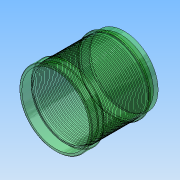
# Autodesk Inventor part: Signal_tower_D
Saved by Autodesk Inventor 2017.3 (Build 213256000, 256)
## iProperties
Created: 2017-03-21
Part Number: Signal_tower_D
Material: Polykarbonát, Čirý
Document SubType Name: Modeling
Designer: CAD
Mass: 43.1519 g
Surface Area: 356.955 cm^2
Volume: 35.9599 cm^3
Density: 1.2 g/cm^3
Appearance: LED – zelená – zap.
Stock Number: SIEMENS
Hmotnost: 0
Hotovo: 0
Objem: 0
X: 0
Y: 0
Z: 0
Author: CAD
Autodesk Inventor part; units mm, degrees
ref_plane "YZ Plane" through (0, 0, 0) normal (1, 0, 0) x (0, 1, 0)
ref_plane "XZ Plane" through (0, 0, 0) normal (0, 1, 0) x (-1, 0, 0)
ref_plane "XY Plane" through (0, 0, 0) normal (0, 0, 1) x (1, 0, 0)
sketch "Náčrt2" plane through (0, 0, 0) normal (0, 0, 1) x (1, 0, 0)
  line L0 (0, 0) -> (-32.5, 0) construction
  line L1 (-32.5, 0) -> (-32.5, 9)
  line L2 (-32.5, 9) -> (-31, 9)
  line L3 (-31, 9) -> (-31, 63)
  line L4 (0, 0) -> (0, 63) construction
  line L5 (-32.5, 0) -> (-35, 0)
  line L6 (-35, 0) -> (-35, 12)
  line L7 (-35, 12) -> (-33, 12)
  line L8 (-33, 12) -> (-33, 55)
  line L9 (-33, 55) -> (-34.5, 55)
  line L10 (-34.5, 55) -> (-34.5, 57)
  line L11 (-34.5, 57) -> (-32.5, 57)
  line L12 (-32.5, 57) -> (-32.5, 66)
  line L13 (-32.5, 66) -> (0, 66)
  line L14 (0, 66) -> (0, 63)
  line L15 (0, 63) -> (-31, 63)
  dimension "d0" = 65
  dimension "d1" = 9
  dimension "d2" = 62
  dimension "d3" = 70
  dimension "d4" = 12
  dimension "d5" = 66
  dimension "d6" = 55
  dimension "d7" = 2
  dimension "d8" = 66
  dimension "d9" = 65
  dimension "d10" = 3
  dimension "d11" = 69
  dimension "d12" = 9
  constraints: 32 end point, 7 perpendicular, 5 horizontal, 4 vertical
  measures "d0" diameter of L1 L4
  measures "d1" distance between parallel lines of L2 L0
  measures "d2" diameter of L3 L4
  measures "d3" diameter of L6 L4
  measures "d4" distance between parallel lines of L7 L5
  measures "d5" diameter of L8 L4
  measures "d6" distance between parallel lines of L9 L0
  measures "d7" distance between parallel lines of L11 L9
  measures "d8" distance between parallel lines of L13 L5
  measures "d9" diameter of L12 L4
  measures "d10" distance between parallel lines of L15 L13
  measures "d11" diameter of L10 L4
  measures "d12" distance between parallel lines of L11 L13
revolve "Rotace1" add sketch "Náčrt2" angle 360 about axis through (0, 0, 0) along (0, 1, 0)
sketch "Náčrt3" plane through (0, 0, 0) normal (0, 0, 1) x (1, 0, 0)
  circle A0 centre (-33.25, 14.5) radius 0.75
  line L0 (35, 12) -> (-35, 12) projected
  line L1 (34.5, 55) -> (-34.5, 55) projected
  line L2 (0, -11) -> (0, 66) projected
  line L3 (-32.5, 16.4967) -> (-32.5, 12.9176) construction
  line L4 (0, 0) -> (0, -18.5925) construction
  circle A1 centre (-33.25, 17) radius 0.75
  circle A2 centre (-33.25, 19.5) radius 0.75
  circle A3 centre (-33.25, 22) radius 0.75
  circle A4 centre (-33.25, 24.5) radius 0.75
  circle A5 centre (-33.25, 27) radius 0.75
  circle A6 centre (-33.25, 29.5) radius 0.75
  circle A7 centre (-33.25, 32) radius 0.75
  circle A8 centre (-33.25, 34.5) radius 0.75
  circle A9 centre (-33.25, 37) radius 0.75
  circle A10 centre (-33.25, 39.5) radius 0.75
  circle A11 centre (-33.25, 42) radius 0.75
  circle A12 centre (-33.25, 44.5) radius 0.75
  circle A13 centre (-33.25, 47) radius 0.75
  circle A14 centre (-33.25, 49.5) radius 0.75
  circle A15 centre (-33.25, 52) radius 0.75
  dimension "d14" = 1.5
  dimension "d15" = 2.5
  dimension "d28" = 65
  dimension "d31" = 2.5
  constraints: 16 centre point, 4 end point, 2 vertical, 1 point on line, 1 tangent, 30 other
  measures "d14" diameter of A0
  measures "d15" distance from line of A0.centre L0
  measures "d28" diameter of L3 L4
  measures "d31" distance of A0.centre A1.centre
revolve "Rotace2" cut sketch "Náčrt3" angle 360 about axis through (0, -10, 0) along (0, 1, 0)
chamfer "Zkosení1" distance 0.5 angle 45 3 edges at (35, 12, 0) (34.5, 55, 0) (35, 0, 0)
